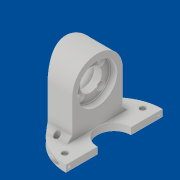
# Autodesk Inventor part: 201-
Saved by Autodesk Inventor 2018 (Build 220112000, 112)
## iProperties
Created: 2020-01-12
Part Number: 201-
Material: Generic
Document SubType Name: Modeling
Designer: Bunny320
Density: 1 g/cm^3
Appearance: Default
Author: Bunny320
## iProperties of the stored document 201-flange-with motor_3DPrint.ipt
Created: 2020-05-08
Part Number: 201-flange-with motor_3DPrint
Material: Generic
Document SubType Name: Modeling
Designer: Bunny320
Density: 1 g/cm^3
Appearance: Default
Author: Bunny320
Autodesk Inventor part; units mm, degrees
ref_plane "YZ Plane" through (0, 0, 0) normal (1, 0, 0) x (0, 1, 0)
ref_plane "XZ Plane" through (0, 0, 0) normal (0, 1, 0) x (-1, 0, 0)
ref_plane "XY Plane" through (0, 0, 0) normal (0, 0, 1) x (1, 0, 0)
sketch "Sketch3" plane through (0, 0, 0) normal (0, 0, 1) x (1, 0, 0)
  circle A0 centre (0, 0) radius 57.5
  dimension "d8" = 115
  constraints: 1 centre point, 1 coincident
  measures "d8" diameter of A0
extrude "Extrusion3" add sketch "Sketch3" along normal blind 8
sketch "Sketch2" plane through (0, 0, 8) normal (0, 0, 1) x (1, 0, 0)
  line L0 (-37, -30) -> (-20, -30)
  line L1 (-20, -30) -> (-20, 30)
  line L2 (-20, 30) -> (-37, 30)
  line L3 (-37, 30) -> (-37, -30)
  line L4 (-37, -30) -> (-20, 30) construction
  line L5 (-20, -30) -> (-37, 30) construction
  point P0 (0, 0)
  point P1 (-28.5, 0)
  dimension "d3" = 17
  dimension "d4" = 60
  dimension "d5" = 20
  constraints: 12 end point, 2 midpoint, 2 parallel, 1 horizontal, 1 perpendicular
  measures "d3" distance of L1.end L2.end
  measures "d4" distance of L2.end L0.start
  measures "d5" distance from line of point (0, 0) L1
extrude "Extrusion2" add sketch "Sketch2" along normal blind 76
full round fillet "Fillet1" first side at (-31.3333, -30, 33.3333) centre faces at (-25.6667, 10, 84) second side at (-25.6667, 30, 33.3333)
sketch "Sketch5" plane through (0, 0, 0) normal (0, 1, 0) x (-1, 0, 0)
  line L0 (37, 53) -> (17.1258, 53)
  line L1 (37, 66) -> (28, 66)
  line L2 (28, 66) -> (28, 75.5)
  line L3 (28, 75.5) -> (27, 75.5)
  line L4 (27, 75.5) -> (27, 76.5)
  line L5 (27, 76.5) -> (20, 76.5)
  line L6 (57.5, 8) -> (-57.5, 8) projected
  line L7 (37, 53) -> (20, 53)
  line L8 (37, 66) -> (37, 53)
  line L9 (37, 8) -> (37, 54) projected
  line L10 (20, 76.5) -> (20, 53)
  point P0 (0, 0)
  dimension "d12" = 47
  dimension "d14" = 45
  dimension "d15" = 1
  dimension "d16" = 26
  dimension "d84" = 45
  constraints: 18 end point, 4 perpendicular, 2 horizontal, 2 point on line, 2 vertical, 1 collinear
  measures "d12" diameter of L5 L0
  measures "d14" diameter of L3 L0
  measures "d15" distance of L2.end L3.end
  measures "d16" diameter of L1 L0
  measures "d84" distance between parallel lines of L6 L0
revolve "Revolution1" cut sketch "Sketch5" angle 360 about axis through (-37, 0, 53) along (1, 0, 0)
sketch "Sketch6" plane through (-28, 0, 53) normal (1, 0, 0) x (0, 0, -1)
  line L0 (-12.3744, -12.3744) -> (12.3744, -12.3744)
  line L1 (12.3744, -12.3744) -> (12.3744, 12.3744)
  line L2 (12.3744, 12.3744) -> (-12.3744, 12.3744)
  line L3 (-12.3744, 12.3744) -> (-12.3744, -12.3744)
  line L4 (-12.3744, -12.3744) -> (12.3744, 12.3744) construction
  line L5 (12.3744, -12.3744) -> (-12.3744, 12.3744) construction
  point P0 (53, 0)
  point P1 (0, 0)
  dimension "d17" = 35
  constraints: 12 end point, 4 coincident, 2 midpoint, 2 parallel, 2 perpendicular, 1 horizontal
  measures "d17" distance of L0.start L1.end
hole "Hole1" at (-28, 12.3744, 65.3744) at (-28, 12.3744, 40.6256) at (-28, -12.3744, 40.6256) at (-28, -12.3744, 65.3744) direction (-1, 0, 0) diameter 4.5 end through all countersink diameter 10 countersink angle 90 clearance for "Countersunk Flat Head Hex Socket Screw DIN EN ISO 10642" size "M4" standard "DIN"
sketch "Sketch7" plane through (0, 0, 8) normal (0, 0, 1) x (1, 0, 0)
  line L0 (-12.4233, 46.3644) -> (0, 0)
  line L1 (0, 80.5) -> (0, -80.5) projected
  dimension "d25" = 48
  dimension "d26" = 15
  constraints: 2 end point
  measures "d25" distance of L0.start L0.end
  measures "d26" angle of L1 L0
hole "Hole2" at (-12.4233, 46.3644, 8) direction (0, 0, -1) diameter 3.4 end through all counterbore diameter 6.5 counterbore depth 3.4 clearance for "Socket Head Cap Screw DIN EN ISO 4762" size "M3" standard "DIN"
pattern_circular "Circular Pattern1" count 12 over 360 about axis through (0, 0, -10) along (0, 0, 1) of "Hole2" skipped copies 3 4 7 8 9 10 11 12 13 14 15 16
sketch "Sketch8" plane through (0, 0, 8) normal (0, 0, 1) x (1, 0, 0)
  line L0 (0, 23.094) -> (20, 11.547)
  line L1 (20, 11.547) -> (20, -11.547)
  line L2 (20, -11.547) -> (0, -23.094)
  line L3 (0, -23.094) -> (-20, -11.547)
  line L4 (-20, -11.547) -> (-20, 11.547)
  line L5 (-20, 11.547) -> (0, 23.094)
  circle A0 centre (0, 0) radius 20
  dimension "d37" = 40
  constraints: 12 end point, 2 coincident, 1 centre point, 13 other
  measures "d37" distance between parallel lines of L1 L4
extrude "Extrusion4" cut sketch "Sketch8" against normal through all contours A0
sketch "Sketch9" plane through (0, 0, 0) normal (0, 0, 1) x (1, 0, 0)
  line L0 (0, 60.5186) -> (63.6838, 60.5186)
  line L1 (63.6838, 60.5186) -> (63.6838, -58.7461)
  line L2 (63.6838, -58.7461) -> (0, -58.7461)
  line L3 (0, -58.7461) -> (0, 60.5186)
  point P0 (0, 0)
  constraints: 8 end point, 2 parallel, 1 horizontal, 1 perpendicular
extrude "Extrusion5" cut sketch "Sketch9" along normal through all
chamfer "Chamfer1" [suppressed]
fillet "Fillet3" [suppressed]
sketch "Sketch10" plane through (-37, 0, 54) normal (-1, 0, 0) x (0, 0, 1)
  line L0 (-54, 57.5) -> (-54, -57.5) projected
  line L1 (-54, -57.5) -> (-46, -57.5) projected
  line L2 (-46, 57.5) -> (-54, 57.5) projected
  line L3 (-47, 51.7679) -> (-50, 50.0359)
  line L4 (-50, 50.0359) -> (-53, 51.7679)
  line L5 (-53, 51.7679) -> (-53, 55.2321)
  line L6 (-53, 55.2321) -> (-50, 56.9641)
  line L7 (-50, 56.9641) -> (-47, 55.2321)
  line L8 (-47, 55.2321) -> (-47, 51.7679)
  point P0 (-54, 0)
  point P1 (-50, 53.5)
  point P2 (-50, -53.5)
  point P3 (-50, 53.5)
  dimension "d55" = 4
  dimension "d56" = 4
  dimension "d57" = 4
  dimension "d58" = 4
  dimension "d67" = 6
  constraints: 12 end point, 1 coincident, 1 vertical, 13 other
  measures "d55" distance from line of L0 point (-50, -53.5)
  measures "d56" distance from line of L1 point (-50, -53.5)
  measures "d57" distance from line of L2 point (-50, 53.5)
  measures "d58" distance from line of L0 point (-50, 53.5)
  measures "d67" distance between parallel lines of L5 L8
hole "Hole4" at (-37, -53.5, 4) direction (1, 0, 0) diameter 3.4 end through all counterbore diameter 6.5 counterbore depth 30 clearance for "Socket Head Cap Screw DIN EN ISO 4762" size "M3" standard "DIN"
hole "Hole5" at (-37, 53.5, 4) direction (1, 0, 0) diameter 3.4 end through all clearance for "Countersunk Flat Head Screw DIN EN ISO 2009" size "M3" standard "DIN"
extrude "Extrusion6" cut sketch "Sketch10" against normal blind 30
sketch "Sketch12" plane through (-37, -30, 8) normal (-1, 0, 0) x (0, 0, 1)
  circle A0 centre (45, 30) radius 13 projected
  circle A1 centre (45, 30) radius 21.1
  arc A2 (46, 0) -> (46, 60) centre (46, 30) ccw projected
  line L0 (0, 0) -> (46, 0) projected
  line L1 (0, 60) -> (46, 60) projected
  line L2 (0, 0) -> (0, 60) projected
  point P0 (-8, 30)
  dimension "d79" = 42.2
  constraints: 1 centre point, 1 coincident
  measures "d79" diameter of A1
extrude "Extrusion7" add sketch "Sketch12" along normal up to surface contours L0 L2 L1 A2 round surface about axis through (0, 0, 0) along (0, 0, 1) radius 57.5 far side no
chamfer "Chamfer2" distance 6 angle 45 2 edges at (-34.5268, -30, 8) (-34.5268, 30, 8)
equation "\"d55\" = 0.5 * d9"
equation "\"d56\" = 0.5 * d9"
equation "\"d57\" = 0.5 * d9"
equation "\"d58\" = 0.5 * d9"
equation "\"d9\" = 8"
body "Solid1"
